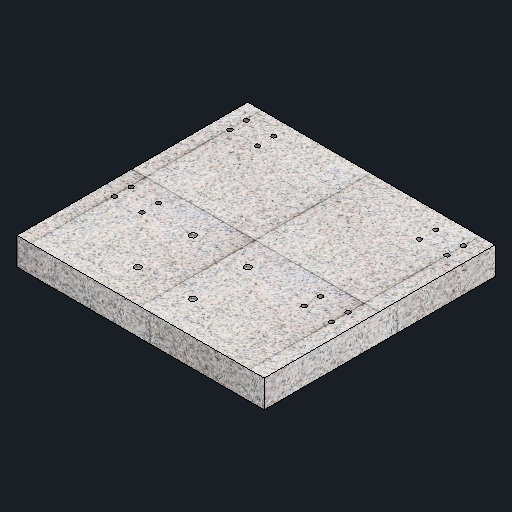
# Autodesk Inventor part: KN-00-01-01
Saved by Autodesk Inventor 2025.2 (Build 292293000, 293)
## iProperties
Created: 2025-01-15
Part Number: KN-00-01-01
Material: Granite, Cut, Polished
Document SubType Name: Modeling
Designer: Kacper Mik
Density: 2.7 g/cm^3
Appearance: Granite - Square Stacked Polished
Mass: 21589 g
Surface Area: 4013.57 cm^2
Volume: 7995.93 cm^3
Author: Kacper Mik
Autodesk Inventor part; units mm, degrees
ref_plane "YZ Plane" through (0, 0, 0) normal (1, 0, 0) x (0, 1, 0)
ref_plane "XZ Plane" through (0, 0, 0) normal (0, 1, 0) x (-1, 0, 0)
ref_plane "XY Plane" through (0, 0, 0) normal (0, 0, 1) x (1, 0, 0)
sketch "Sketch1" plane through (0, 0, 0) normal (0, 1, 0) x (-1, 0, 0)
  line L0 (225, 210) -> (-225, 210)
  line L1 (-225, 210) -> (-225, -210)
  line L2 (-225, -210) -> (225, -210)
  line L3 (225, -210) -> (225, 210)
  line L4 (225, -210) -> (-225, 210) construction
  point P0 (0, 0)
  point P1 (0, 0)
  dimension "d0" = 450
  dimension "d1" = 420
  constraints: 10 end point, 2 parallel, 1 coincident, 1 horizontal, 1 midpoint, 1 perpendicular
  measures "d0" distance of L2.end L1.end
  measures "d1" distance of L1.end L0.end
extrude "plyta" add sketch "Sketch1" along normal blind 50
sketch "Sketch3" plane through (0, 0, 0) normal (0, -1, 0) x (1, 0, 0)
  line L0 (225, -210) -> (-225, -210) projected
  line L1 (225, 210) -> (225, -210) projected
  line L2 (-225, -210) -> (-225, 0) projected
  line L3 (0, 210) -> (225, 210) projected
  point P0 (0, 0)
  point P1 (-175, -160)
  point P2 (175, -160)
  point P3 (-175, 160)
  point P4 (175, 160)
  dimension "d18" = 50
  dimension "d19" = 50
  dimension "d20" = 50
  dimension "d21" = 50
  constraints: 2 horizontal alignment, 2 vertical alignment
  measures "d18" distance from line of L0 point (175, -160)
  measures "d19" distance from line of L1 point (175, -160)
  measures "d20" distance from line of L2 point (-175, 160)
  measures "d21" distance from line of L3 point (-175, 160)
hole "Hole2" at (-175, 0, -160) at (175, 0, -160) at (-175, 0, 160) at (175, 0, 160) direction (0, 1, 0) diameter 12 depth 9
sketch "Sketch4" plane through (0, 50, 0) normal (0, 1, 0) x (1, 0, 0)
  line L0 (0, 294) -> (0, -294) construction
  line L1 (-225, -210) -> (225, -210) construction
  point P0 (0, 0)
  point P1 (-65, -150)
  point P2 (35, -150)
  point P3 (-65, -50)
  point P4 (35, -50)
  dimension "d29" = 60
  dimension "d30" = 100
  dimension "d32" = 100
  dimension "d40" = 35
  constraints: 2 horizontal alignment, 2 vertical alignment
  measures "d29" distance from line of L1 point (35, -150)
  measures "d30" distance of point (35, -150) point (-65, -150)
  measures "d32" distance of point (-65, -150) point (-65, -50)
  measures "d40" distance from line of L0 point (35, -150)
hole "Hole3" at (-65, 50, 150) at (35, 50, 150) at (-65, 50, 50) at (35, 50, 50) direction (0, -1, 0) diameter 12 depth 9
sketch "Sketch5" plane through (0, 50, 0) normal (0, 1, 0) x (1, 0, 0)
  circle A0 centre (197.5, -60) radius 5.75 construction
  circle A1 centre (147.5, -30) radius 5.75 construction
  line L0 (195, 80) -> (215, 80) construction
  line L1 (195, -12.5491) -> (195, 80) construction
  line L2 (150, -12.5491) -> (195, -12.5491) construction
  line L3 (150, 80) -> (150, -12.5491) construction
  line L4 (130, 80) -> (150, 80) construction
  line L5 (130, -80) -> (130, 80) construction
  line L6 (215, -80) -> (130, -80) construction
  line L7 (215, -80) -> (215, 80) construction
  circle A2 centre (147.5, -60) radius 5.75 construction
  circle A3 centre (197.5, -30) radius 5.75 construction
  circle A4 centre (147.5, 150) radius 5.75 construction
  circle A5 centre (197.5, 180) radius 5.75 construction
  line L8 (215, 130) -> (130, 130) construction
  line L9 (215, 130) -> (215, 200) construction
  line L10 (130, 200) -> (215, 200) construction
  line L11 (130, 130) -> (130, 200) construction
  circle A6 centre (147.5, 180) radius 5.75 construction
  circle A7 centre (197.5, 150) radius 5.75 construction
  point P0 (0, 0)
  constraints: 8 coincident
hole "Hole4" at (147.5, 50, 60) at (147.5, 50, 30) at (147.5, 50, -150) at (147.5, 50, -180) at (197.5, 50, -180) at (197.5, 50, -150) at (197.5, 50, 30) at (197.5, 50, 60) direction (0, -1, 0) diameter 8.376 end through all thread size "M10x1.5" class "6H" standard "ISO Metric profile"
mirror "Mirror1" about plane through (0, 0, 0) normal (1, 0, 0) of "Hole4"
equation "\"d20\" = d19"
equation "\"d21\" = d18"
body "Solid1"
